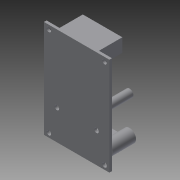
# Autodesk Inventor part: step driver
Saved by Autodesk Inventor 2015 (Build 190159000, 159)
## iProperties
Created: 2015-05-04
Part Number: step driver
Material: Ogólny
Document SubType Name: Modeling
Designer: Kuba
Density: 1 g/cm^3
Appearance: Domyślna
Author: Kuba
Autodesk Inventor part; units mm, degrees
ref_plane "YZ Plane" through (0, 0, 0) normal (1, 0, 0) x (0, 1, 0)
ref_plane "XZ Plane" through (0, 0, 0) normal (0, 1, 0) x (-1, 0, 0)
ref_plane "XY Plane" through (0, 0, 0) normal (0, 0, 1) x (1, 0, 0)
sketch "Szkic1" plane through (0, 0, 0) normal (0, 1, 0) x (-1, 0, 0)
  line L0 (-25.25, -37.75) -> (25.25, -37.75)
  line L1 (25.25, -37.75) -> (25.25, 37.75)
  line L2 (25.25, 37.75) -> (-25.25, 37.75)
  line L3 (-25.25, 37.75) -> (-25.25, -37.75)
  line L4 (-25.25, -37.75) -> (25.25, 37.75) construction
  line L5 (25.25, -37.75) -> (-25.25, 37.75) construction
  point P0 (0, 0)
  dimension "d0" = 50.5
  dimension "d1" = 75.5
  constraints: 12 end point, 2 midpoint, 2 parallel, 1 horizontal, 1 perpendicular
  measures "d0" distance of L2.end L1.end
  measures "d1" distance of L1.end L0.end
extrude "Wyciągnięcie proste1" add sketch "Szkic1" along normal blind 2
sketch "Szkic2" plane through (0, 2, 0) normal (0, 1, 0) x (1, 0, 0)
  line L0 (25.25, 37.75) -> (-25.25, 37.75) projected
  line L1 (-25.25, 37.75) -> (-25.25, -37.75) projected
  line L2 (-25.25, -37.75) -> (25.25, -37.75) projected
  line L3 (25.25, -37.75) -> (25.25, 37.75) projected
  line L4 (-25.25, 37.75) -> (-25.25, -37.75) projected
  point P0 (0, 0)
  point P1 (-21.5, -34.5)
  point P2 (-21.5, 34.5)
  point P3 (21.5, 34.5)
  point P4 (21.5, -34.5)
  point P5 (-15.25, 14.5)
  point P6 (15.25, 14.5)
  dimension "d4" = 69
  dimension "d5" = 69
  dimension "d6" = 43
  dimension "d7" = 43
  dimension "d8" = 75.5
  dimension "d9" = 50.5
  dimension "d10" = 3.75
  dimension "d11" = 3.25
  dimension "d13" = 3.75
  dimension "d14" = 3.25
  dimension "d15" = 20
  dimension "d16" = 20
  dimension "d17" = 30.5
  dimension "d19" = 10
  dimension "d20" = 10
  measures "d4" distance of point (-21.5, 34.5) point (-21.5, -34.5)
  measures "d5" distance of point (21.5, 34.5) point (21.5, -34.5)
  measures "d6" distance of point (21.5, -34.5) point (-21.5, -34.5)
  measures "d7" distance of point (21.5, 34.5) point (-21.5, 34.5)
  measures "d8" distance of L0.end L1.end
  measures "d9" distance of L1.end L2.end
  measures "d10" distance from line of point (-21.5, -34.5) L1
  measures "d11" distance from line of L2 point (-21.5, -34.5)
  measures "d13" distance from line of L1 point (-21.5, 34.5)
  measures "d14" distance from line of L2 point (21.5, -34.5)
  measures "d15" vertical distance of point (-21.5, 34.5) point (-15.25, 14.5)
  measures "d16" vertical distance of point (21.5, 34.5) point (15.25, 14.5)
  measures "d17" distance of point (-15.25, 14.5) point (15.25, 14.5)
  measures "d19" distance from line of L1 point (-15.25, 14.5)
  measures "d20" distance from line of L3 point (15.25, 14.5)
hole "Otwór1" at (-21.5, 2, 34.5) at (-21.5, 2, -34.5) at (21.5, 2, -34.5) at (21.5, 2, 34.5) at (-15.25, 2, -14.5) at (15.25, 2, -14.5) direction (0, -1, 0) diameter 3.5 end through all
sketch "Szkic3" plane through (0, 2, 0) normal (0, 1, 0) x (1, 0, 0)
  circle A0 centre (-15.25, 14.5) radius 1.75 projected
  circle A1 centre (21.5, 34.5) radius 1.75 projected
  circle A2 centre (-21.5, -34.5) radius 1.75 projected
  circle A3 centre (-21.5, 34.5) radius 1.75 projected
  circle A4 centre (21.5, -34.5) radius 1.75 projected
  circle A5 centre (15.25, 14.5) radius 1.75 projected
  line L0 (25.25, 37.75) -> (-25.25, 37.75) projected
  line L1 (-25.25, 37.75) -> (-25.25, -37.75) projected
  line L2 (-25.25, -37.75) -> (25.25, -37.75) projected
  line L3 (25.25, -37.75) -> (25.25, 37.75) projected
  line L4 (-15.25, 37.75) -> (15.25, 37.75)
  line L5 (15.25, 37.75) -> (15.25, 27.25)
  line L6 (15.25, 27.25) -> (-15.25, 27.25)
  line L7 (-15.25, 27.25) -> (-15.25, 37.75)
  circle A6 centre (20.8161, 25.0959) radius 5
  line L8 (-15.25, -37.75) -> (15.25, -37.75)
  line L9 (15.25, -37.75) -> (15.25, -27.25)
  line L10 (15.25, -27.25) -> (-15.25, -27.25)
  line L11 (-15.25, -27.25) -> (-15.25, -37.75)
  line L12 (-25.25, -27.25) -> (-15.25, -27.25)
  line L13 (-15.25, -27.25) -> (-15.25, 7.75)
  line L14 (-15.25, 7.75) -> (-25.25, 7.75)
  line L15 (-25.25, 7.75) -> (-25.25, -27.25)
  circle A7 centre (20.8161, -3.2547) radius 3
  point P0 (0, 0)
  dimension "d28" = 10.5
  dimension "d29" = 10
  dimension "d30" = 10
  dimension "d31" = 10
  dimension "d32" = 10.5
  dimension "d33" = 10
  dimension "d34" = 10
  dimension "d35" = 35
  dimension "d36" = 6
  constraints: 24 end point, 6 parallel, 3 horizontal, 3 perpendicular, 3 point on line, 2 centre point
  measures "d28" distance of L4.end L5.end
  measures "d29" distance between parallel lines of L1 L7
  measures "d30" distance between parallel lines of L5 L3
  measures "d31" diameter of A6
  measures "d32" distance of L9.end L8.end
  measures "d33" distance between parallel lines of L1 L11
  measures "d34" distance between parallel lines of L9 L3
  measures "d35" distance of L13.end L12.end
  measures "d36" diameter of A7
extrude "Wyciągnięcie proste2" add sketch "Szkic3" along normal blind 18 contours L5 L6 L7 L0 | A6 L3 | L3 A6 | L2 L11 L10 L9 | A7
sketch "Szkic4" plane through (0, 2, 0) normal (0, 1, 0) x (1, 0, 0)
  line L0 (15.25, -27.25) -> (15.25, -37.75) projected
  line L1 (15.25, -37.75) -> (25.25, -37.75) projected
  line L2 (25.25, -37.75) -> (25.25, 22.7849) projected
  arc A0 (25.25, 27.4069) -> (25.25, 22.7849) centre (20.8161, 25.0959) ccw projected
  line L3 (25.25, 27.4069) -> (25.25, 37.75) projected
  line L4 (25.25, 37.75) -> (15.25, 37.75) projected
  line L5 (15.25, 37.75) -> (15.25, 27.25) projected
  line L6 (15.25, 27.25) -> (-15.25, 27.25) projected
  line L7 (-15.25, 27.25) -> (-15.25, 37.75) projected
  line L8 (-15.25, 37.75) -> (-25.25, 37.75) projected
  line L9 (-25.25, 37.75) -> (-25.25, -37.75) projected
  line L10 (-25.25, -37.75) -> (-15.25, -37.75) projected
  line L11 (-15.25, -37.75) -> (-15.25, -27.25) projected
  line L12 (-15.25, -27.25) -> (15.25, -27.25) projected
  circle A1 centre (20.8161, -3.2547) radius 3 projected
  circle A2 centre (-15.25, 14.5) radius 1.75 projected
  circle A3 centre (21.5, 34.5) radius 1.75 projected
  circle A4 centre (-21.5, -34.5) radius 1.75 projected
  circle A5 centre (-21.5, 34.5) radius 1.75 projected
  circle A6 centre (21.5, -34.5) radius 1.75 projected
  circle A7 centre (15.25, 14.5) radius 1.75 projected
  line L13 (-25.25, 37.75) -> (-25.25, -37.75) projected
  line L14 (-25.25, -27.25) -> (-14.25, -27.25)
  line L15 (-14.25, -27.25) -> (-14.25, 7.75)
  line L16 (-14.25, 7.75) -> (-25.25, 7.75)
  line L17 (-25.25, 7.75) -> (-25.25, -27.25)
  point P0 (0, 0)
  dimension "d39" = 11
  dimension "d40" = 35
  constraints: 8 end point, 2 parallel, 1 horizontal, 1 perpendicular, 1 point on line
  measures "d39" distance of L16.end L15.end
  measures "d40" distance of L15.end L14.end
extrude "Wyciągnięcie proste3" add sketch "Szkic4" along normal blind 6 contours L12 L14 L9 L16 L15
sketch "Szkic5" plane through (0, 0, 0) normal (0, -1, 0) x (1, 0, 0)
  circle A0 centre (-15.25, -14.5) radius 1.75 projected
  circle A1 centre (21.5, -34.5) radius 1.75 projected
  circle A2 centre (-21.5, 34.5) radius 1.75 projected
  circle A3 centre (-21.5, -34.5) radius 1.75 projected
  circle A4 centre (21.5, 34.5) radius 1.75 projected
  circle A5 centre (15.25, -14.5) radius 1.75 projected
  line L0 (25.25, -37.75) -> (-25.25, -37.75) projected
  line L1 (25.25, 37.75) -> (25.25, -37.75) projected
  line L2 (-25.25, 37.75) -> (25.25, 37.75) projected
  line L3 (-25.25, -37.75) -> (-25.25, 37.75) projected
  line L4 (-18, -7.5) -> (18, -7.5)
  line L5 (18, -21.5) -> (-18, -21.5)
  arc A6 (-15.25, -17.25) -> (-15.25, -11.75) centre (-15.25, -14.5) ccw
  arc A7 (15.25, -11.75) -> (15.25, -17.25) centre (15.25, -14.5) ccw
  line L6 (-15.25, -11.75) -> (-18, -11.75)
  line L7 (-15.25, -17.25) -> (-18, -17.25)
  line L8 (15.25, -11.75) -> (18, -11.75)
  line L9 (15.25, -17.25) -> (18, -17.25)
  line L10 (-18, -21.5) -> (-18, -17.25)
  line L11 (-18, -11.75) -> (-18, -7.5)
  line L12 (18, -7.5) -> (18, -11.75)
  line L13 (18, -17.25) -> (18, -21.5)
  point P0 (0, 0)
  dimension "d43" = 36
  dimension "d44" = 14
  dimension "d45" = 7
  dimension "d46" = 7
  constraints: 20 end point, 6 perpendicular, 5 parallel, 4 point on circle, 4 point on line, 2 centre point, 2 coincident, 1 horizontal
  measures "d43" distance of L4.start L4.end
  measures "d44" distance of L5.end L4.start
  measures "d45" distance from line of L4 A0.centre
  measures "d46" distance from line of L5 A0.centre
extrude "Wyciągnięcie proste4" add sketch "Szkic5" along normal blind 5 contours L4 L12 L8 A7 L9 L13 L5 L10 L7 A6 L6 L11
equation "\"d5\" = d4"
equation "\"d7\" = d6"
equation "\"d10\" = -0.5 * d6 + 0.5 * d9"
equation "\"d11\" = -0.5 * d4 + 0.5 * d8"
equation "\"d13\" = d10"
equation "\"d14\" = d11"
equation "\"d16\" = d15"
equation "\"d19\" = d20"
equation "\"d30\" = d29"
equation "\"d34\" = d33"
equation "\"d45\" = d46"
equation "\"d47\" = d48"
equation "\"d48\" = 2.75"
